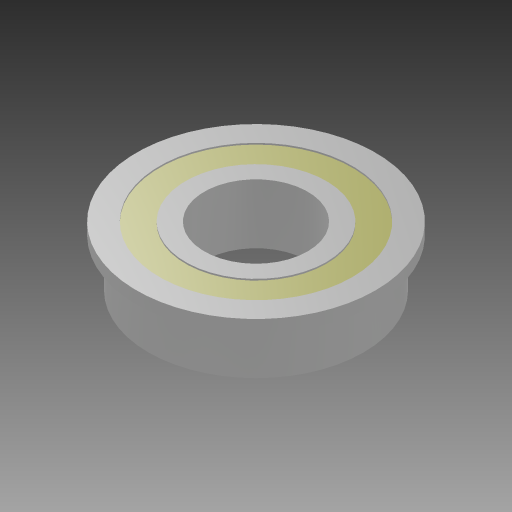
# Autodesk Inventor part: 217-4006
Saved by Autodesk Inventor 2023 (Build 270158000, 158)
## iProperties
Created: 2020-11-14
Material: Steel
Document SubType Name: Modeling
Density: 7.85 g/cm^3
Appearance: Anodized - Light Gray
Part Number: 217-4006
Mass: 31.8165 g
Surface Area: 24.1286 cm^2
Volume: 4.05306 cm^3
Revision Number: 0
Autodesk Inventor part; units mm, degrees
ref_plane "YZ Plane" through (0, 0, 0) normal (1, 0, 0) x (0, 1, 0)
ref_plane "XZ Plane" through (0, 0, 0) normal (0, 1, 0) x (-1, 0, 0)
ref_plane "XY Plane" through (0, 0, 0) normal (0, 0, 1) x (1, 0, 0)
sketch "Sketch15" plane through (0, 0, 0) normal (0, 0, 1) x (1, 0, 0)
  line L0 (0, 0) -> (0, 6.6558) construction
  line L1 (0, 0) -> (6.875, 3.9688) construction
  line L2 (6.875, 3.9688) -> (6.875, -3.9688)
  line L3 (6.875, -3.9688) -> (0, 0) construction
  line L4 (6.875, 3.9688) -> (9.3458, 3.9688)
  line L5 (9.3458, 3.9688) -> (9.3458, 3.6433)
  line L6 (9.3458, 3.6433) -> (12.805, 3.6433)
  line L7 (12.805, 3.6433) -> (12.805, 3.9688)
  line L8 (12.805, 3.9688) -> (15.875, 3.9688)
  line L9 (15.875, 3.9688) -> (15.875, 2.3939)
  line L10 (15.875, 2.3939) -> (14.2875, 2.3939)
  line L11 (14.2875, 2.3939) -> (14.2875, -3.9688)
  line L12 (14.2875, -3.9688) -> (12.805, -3.9688)
  line L13 (12.805, -3.9688) -> (12.805, -3.6433)
  line L14 (12.805, -3.6433) -> (9.3458, -3.6433)
  line L15 (9.3458, -3.6433) -> (9.3458, -3.9688)
  line L16 (9.3458, -3.9688) -> (6.875, -3.9688)
  dimension "FlangeOD" = 31.75
  dimension "FlangeThickness" = 1.5748
  dimension "BearingID" = 13.75
  dimension "BearingOD" = 28.575
  dimension "d177" = 7.2866
  dimension "BearingThickness" = 7.9375
  dimension "d179" = 2.4708
  dimension "d180" = 1.4825
  dimension "d181" = 7.4125
  constraints: 34 end point, 10 perpendicular, 4 point on line, 2 collinear, 2 equal length, 2 vertical, 1 horizontal
  measures "FlangeOD" diameter of L9 L0
  measures "FlangeThickness" distance between parallel lines of L10 L8
  measures "BearingID" diameter of L2 L0
  measures "BearingOD" diameter of L11 L0
  measures "d177" distance between parallel lines of L14 L6
  measures "BearingThickness" distance between parallel lines of L12 L8
  measures "d179" distance between parallel lines of L2 L5
  measures "d180" distance between parallel lines of L11 L7
  measures "d181" distance between parallel lines of L11 L2
revolve "Revolution1" add sketch "Sketch15" angle 360 about axis through (0, 0, 0) along (0, 1, 0)
sketch "Sketch17" plane through (0, 3.9687, 0) normal (0, 1, 0) x (1, 0, 0)
  circle A0 centre (0, 0) radius 6.875 projected
  line L0 (-7.9386, 0) -> (-3.9693, 6.875)
  line L1 (-3.9693, 6.875) -> (3.9693, 6.875)
  line L2 (3.9693, 6.875) -> (7.9386, 0)
  line L3 (7.9386, 0) -> (3.9693, -6.875)
  line L4 (3.9693, -6.875) -> (-3.9693, -6.875)
  line L5 (-3.9693, -6.875) -> (-7.9386, 0)
  point P0 (0, 0)
  constraints: 12 end point, 1 coincident, 1 horizontal, 1 tangent, 13 other
extrude "Hex" [suppressed]
sketch "Sketch16" plane through (0, 3.6433, 0) normal (0, 1, 0) x (1, 0, 0)
  circle A0 centre (0, 0) radius 9.3458 projected
  circle A1 centre (0, 0) radius 12.805 projected
extrude "Shielded" add sketch "Sketch16" along normal blind 0.127
mirror "Shielded Mirror" about plane through (0, 0, 0) normal (0, 1, 0) of "Shielded"
sketch "Sketch18" plane through (0, 3.6433, 0) normal (0, 1, 0) x (1, 0, 0)
  circle A0 centre (0, 0) radius 2.6458 projected
  circle A1 centre (0, 0) radius 4.1275 projected
extrude "Sealed" [suppressed]
mirror "Sealed Mirror" [suppressed]
equation "\"pi\" = 3.141593"
body "Solid1"
